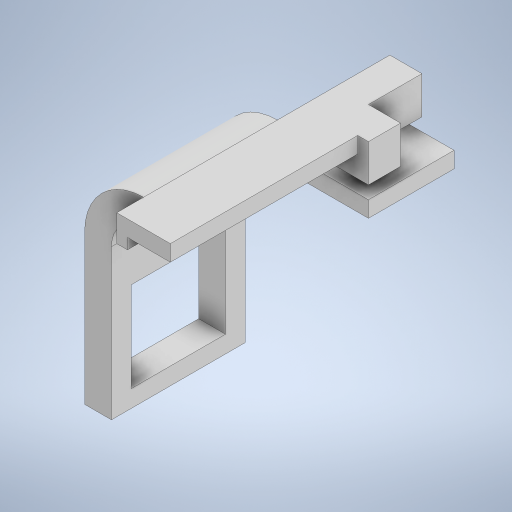
# Autodesk Inventor part: camera_zig
Saved by Autodesk Inventor 2024 (Build 280153000, 153)
## iProperties
Created: 2024-06-11
Part Number: camera_zig
Material: 一般
Document SubType Name: Modeling
Designer: Akio
Density: 1 g/cm^3
Appearance: 既定
Author: Akio
Autodesk Inventor part; units mm, degrees
ref_plane "YZ Plane" through (0, 0, 0) normal (1, 0, 0) x (0, 1, 0)
ref_plane "XZ Plane" through (0, 0, 0) normal (0, 1, 0) x (-1, 0, 0)
ref_plane "XY Plane" through (0, 0, 0) normal (0, 0, 1) x (1, 0, 0)
sketch "スケッチ1" plane through (0, 0, 0) normal (0, 1, 0) x (-1, 0, 0)
  line L0 (0, 0) -> (-4, 0)
  line L1 (-4, 0) -> (-4, -17.5)
  line L2 (-4, -17.5) -> (0, -17.5)
  line L3 (0, -17.5) -> (0, 0)
  dimension "d6" = 17.5
  dimension "d7" = 4
  constraints: 8 end point, 2 parallel, 1 horizontal, 1 perpendicular
  measures "d6" distance between parallel lines of L2 L0
  measures "d7" distance from line of L1 L0.start
extrude "押し出し1" add sketch "スケッチ1" along normal blind 1.5
ref_plane "作業平面1" through (0, -2, 0) normal (0, -1, 0) x (1, 0, 0)
sketch "スケッチ2" plane through (0, -2, 0) normal (0, -1, 0) x (1, 0, 0)
  line L0 (4, 0) -> (4, -17.5) projected
  line L1 (4, -17.5) -> (0, -17.5) projected
  line L2 (0, -17.5) -> (0, 0) projected
  line L3 (0, 0) -> (4, 0) projected
  line L4 (0, -17.5) -> (5, -17.5)
  line L5 (5, -17.5) -> (5, -20.5)
  line L6 (5, -20.5) -> (0, -20.5)
  line L7 (0, -20.5) -> (0, -17.5)
  line L8 (0, -20.5) -> (2, -20.5)
  line L9 (2, -20.5) -> (2, -25.5)
  line L10 (2, -25.5) -> (0, -25.5)
  line L11 (0, -25.5) -> (0, -20.5)
  dimension "d9" = 5
  dimension "d10" = 3
  dimension "d11" = 2
  dimension "d12" = 5
  constraints: 16 end point, 4 parallel, 2 horizontal, 2 perpendicular
  measures "d9" distance of L5.end L6.end
  measures "d10" distance of L4.end L5.end
  measures "d11" distance of L9.end L10.end
  measures "d12" distance of L8.end L9.end
extrude "押し出し2" add sketch "スケッチ2" against normal blind 3.5 contours L4 L5 L6 L7 L1 | L6 L9 L10 L11
ref_plane "作業平面2" through (0, -3.2, 0) normal (0, -1, 0) x (1, 0, 0)
sketch "スケッチ3" plane through (0, -3.2, 0) normal (0, -1, 0) x (1, 0, 0)
  line L0 (4, -17.5) -> (5, -17.5) projected
  line L1 (0, -25.5) -> (0, 0) projected
  line L2 (5, -17.5) -> (0, -17.5)
  line L3 (0, -17.5) -> (0, -25.5)
  line L4 (0, -25.5) -> (5, -25.5)
  line L5 (5, -25.5) -> (5, -17.5)
  constraints: 8 end point, 2 parallel, 1 horizontal, 1 perpendicular
extrude "押し出し3" add sketch "スケッチ3" along normal blind 1.5
sketch "スケッチ4" plane through (0, 0, 0) normal (-1, 0, 0) x (0, 0, 1)
  line L0 (-25.5, 1.5) -> (0, 1.5) projected
  line L1 (-25.5, 1.5) -> (-17.5, 1.5)
  line L2 (-17.5, 1.5) -> (-17.5, -4.7)
  line L3 (-17.5, -4.7) -> (-25.5, -4.7)
  line L4 (-25.5, -4.7) -> (-25.5, 1.5)
  point P0 (0, 0)
  constraints: 8 end point, 2 parallel, 1 horizontal, 1 perpendicular
extrude "押し出し4" add sketch "スケッチ4" along normal blind 1
sketch "スケッチ5" plane through (0, 0, -17.5) normal (0, 0, 1) x (1, 0, 0)
  line L0 (2, 1.5) -> (-1, 1.5) projected
  line L1 (0, 1.5) -> (-1, 1.5)
  line L2 (-1, 1.5) -> (-1, -1)
  line L3 (-1, -1) -> (0, -1)
  line L4 (0, -1) -> (0, 1.5)
  line L5 (0, 0) -> (0, 1.5) projected
  point P0 (-1, 1.5)
  dimension "d20" = 1
  dimension "d21" = 2.5
  dimension "d62" = 0
  constraints: 8 end point, 2 parallel, 1 horizontal, 1 perpendicular, 1 point on line
  measures "d20" distance of L3.end L2.end
  measures "d21" distance of L2.end L1.end
  measures "d62" distance between parallel lines of L5 L4
extrude "押し出し5" add sketch "スケッチ5" along normal up to surface (17.5 mm away)
sketch "スケッチ7" plane through (4, 1.5, -17.5) normal (0, 0, 1) x (1, 0, 0)
  arc A0 (-5, -2.5) -> (-8, -5.5) centre (-5, -5.5) ccw
  line L0 (-5, -5.5) -> (-5, -2.5) construction
  line L1 (-5, -5.5) -> (-8, -5.5) construction
  line L2 (-4, -1.5) -> (0, -1.5) projected
  line L3 (-5, -2.5) -> (-5, 0) projected
  arc A1 (-5, 0) -> (-10.5, -5.5) centre (-5, -5.5) ccw
  line L4 (-5, -2.5) -> (-5, -1)
  line L5 (-10.5, -5.5) -> (-8, -5.5)
  dimension "d29" = 3
  dimension "d31" = 90
  dimension "d32" = 4
  dimension "d33" = 0
  dimension "d34" = 5.5
  constraints: 8 end point, 4 point on circle, 2 centre point, 1 coincident, 1 collinear
  measures "d29" radius of A0
  measures "d31" angle of L0 L1
  measures "d32" distance from line of L2 L0.start
  measures "d33" distance between parallel lines of L0 L3
  measures "d34" radius of A1
extrude "押し出し6" add sketch "スケッチ7" along normal up to surface (17.5 mm away)
sketch "スケッチ8" plane through (-6.5, -4, -17.5) normal (0, -1, 0) x (1, 0, 0)
  line L0 (0, 0) -> (0, 17.5) projected
  line L1 (2.5, 0) -> (5.5, 0) projected
  line L2 (0, 17.5) -> (2.5, 17.5)
  line L3 (2.5, 17.5) -> (2.5, 0)
  line L4 (2.5, 0) -> (0, 0)
  line L5 (0, 0) -> (0, 17.5)
  point P0 (6.5, 17.5)
  constraints: 8 end point, 2 parallel, 1 horizontal, 1 perpendicular
extrude "押し出し7" add sketch "スケッチ8" along normal blind 4
sketch "スケッチ9" plane through (-6.5, -8, -17.5) normal (0, -1, 0) x (1, 0, 0)
  line L0 (2.5, 0) -> (2.5, 17.5) projected
  line L1 (0, 0) -> (0, 17.5) projected
  line L2 (2.5, 0) -> (0, 0)
  line L3 (0, 0) -> (0, 17.5)
  line L4 (0, 17.5) -> (2.5, 17.5)
  line L5 (2.5, 17.5) -> (2.5, 0)
  point P0 (6.5, 17.5)
  constraints: 8 end point, 2 parallel, 1 horizontal, 1 perpendicular
extrude "押し出し8" add sketch "スケッチ9" along normal blind 10
sketch "スケッチ11" plane through (-4, -4, 0) normal (1, 0, 0) x (0, 0, -1)
  line L0 (4.35, -4) -> (13.15, -4)
  line L1 (13.15, -4) -> (13.15, -12.4)
  line L2 (13.15, -12.4) -> (4.35, -12.4)
  line L3 (4.35, -12.4) -> (4.35, -4)
  line L4 (0, 0) -> (0, -14) projected
  line L5 (17.5, 0) -> (0, 0) projected
  point P0 (0, 4)
  point P1 (8.75, -4)
  dimension "d50" = 8.8
  dimension "d51" = 8.4
  dimension "d53" = 4
  dimension "d63" = 4.35
  constraints: 8 end point, 2 parallel, 1 horizontal, 1 midpoint, 1 perpendicular
  measures "d50" distance of L1.end L2.end
  measures "d51" distance of L0.end L1.end
  measures "d53" distance between parallel lines of L5 L0
  measures "d63" distance between parallel lines of L4 L3
extrude "押し出し9" cut sketch "スケッチ11" against normal through all
sketch "スケッチ12" plane through (-6.5, -4, -17.5) normal (-1, 0, 0) x (0, 0, 1)
  line L0 (17.5, 0) -> (17.5, -14) projected
  line L1 (17.5, 5.5) -> (0, 5.5) projected
  line L2 (17.5, -14) -> (15, -14)
  line L3 (15, -14) -> (15, 5.5)
  line L4 (15, 5.5) -> (17.5, 5.5)
  line L5 (17.5, 5.5) -> (17.5, -14)
  line L6 (0, -14) -> (17.5, -14) projected
  line L7 (0, -14) -> (2.5, -14)
  line L8 (2.5, -14) -> (2.5, 5.5)
  line L9 (2.5, 5.5) -> (0, 5.5)
  line L10 (0, 5.5) -> (0, -14)
  point P0 (17.5, 4)
  dimension "d56" = 2.5
  dimension "d57" = 2.5
  constraints: 16 end point, 4 parallel, 2 horizontal, 2 perpendicular, 2 point on line
  measures "d56" distance of L3.end L4.end
  measures "d57" distance of L9.end L8.end
extrude "押し出し10" cut sketch "スケッチ12" against normal up to surface (5.5 mm away) contours L0 L2 L3 L1 L5 | L6 L10 L1 L8
fillet "フィレット2" [suppressed]
equation "\"d13\" = t_up_con + bottom_offset"
equation "\"d16\" = t_up_con"
equation "\"d53\" = flat_first"
equation "\"t_up_con\" = 1.5"
equation "\"bottom_offset\" = 2"
equation "\"flat_first\" = 4"
